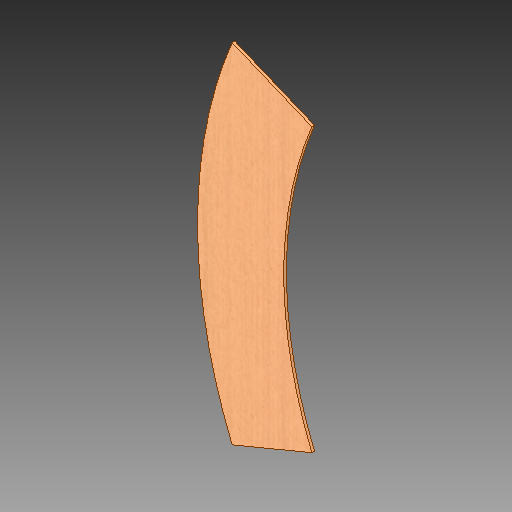
# Autodesk Inventor part: rearformer
Saved by Autodesk Inventor 2019 (Build 230136000, 136)
## iProperties
Created: 2019-01-07
Part Number: rearformer
Material: Wood (Cherry)
Document SubType Name: Modeling
Designer: gaincarlo
Density: 0.63 g/cm^3
Appearance: Cherry - Natural Low Gloss
Author: gaincarlo
Autodesk Inventor part; units mm, degrees
ref_plane "YZ Plane" through (0, 0, 0) normal (1, 0, 0) x (0, 1, 0)
ref_plane "XZ Plane" through (0, 0, 0) normal (0, 1, 0) x (-1, 0, 0)
ref_plane "Work Plane1" through (0, 0, 0) normal (0, 0, 1) x (1, 0, 0)
sketch "Sketch1" plane through (0, 0, 0) normal (0, 0, 1) x (1, 0, 0)
  line L0 (-300, -300) -> (-300, 300) construction
  line L1 (-300, 300) -> (300, 300) construction
  line L2 (300, 300) -> (300, -300) construction
  line L3 (300, -300) -> (-300, -300) construction
  line L4 (-254.3277, 283.4578) -> (-250.5009, 292.6966) construction
  line L5 (-250.5009, 292.6966) -> (303.8268, 63.0866) construction
  line L6 (303.8268, 63.0866) -> (300, 53.8478) construction
  line L7 (300, 53.8478) -> (-254.3277, 283.4578) construction
  line L8 (300, -53.8478) -> (303.8268, -63.0866) construction
  line L9 (303.8268, -63.0866) -> (-250.5009, -292.6966) construction
  line L10 (-250.5009, -292.6966) -> (-254.3277, -283.4578) construction
  line L11 (-254.3277, -283.4578) -> (300, -53.8478) construction
  line L12 (-254.3277, 283.4578) -> (-250.5009, 292.6966) construction
  line L13 (-250.5009, 292.6966) -> (303.8268, 63.0866) construction
  line L14 (303.8268, 63.0866) -> (300, 53.8478) construction
  line L15 (300, 53.8478) -> (-254.3277, 283.4578) construction
  line L16 (300, -53.8478) -> (303.8268, -63.0866) construction
  line L17 (303.8268, -63.0866) -> (-250.5009, -292.6966) construction
  line L18 (-250.5009, -292.6966) -> (-254.3277, -283.4578) construction
  line L19 (-254.3277, -283.4578) -> (300, -53.8478) construction
  arc A0 (34.4092, 161.6757) -> (34.4092, -161.6757) centre (430, 0) ccw construction
  line L20 (35.1767, 163.5412) -> (-57.2112, 201.8095)
  line L21 (35.1767, -163.5412) -> (-57.2112, -201.8095)
  arc A1 (35.1767, 163.5412) -> (35.1767, -163.5412) centre (430, 0) ccw
  arc A2 (-57.2112, 201.8095) -> (-57.2112, -201.8095) centre (430, 0) ccw
  point P0 (0, 0)
  dimension "d2" = 100
  constraints: 44 end point, 4 point on circle, 4 point on line, 2 centre point, 2 coincident, 2 horizontal, 2 vertical, 28 other
  measures "d2" radial gap between concentric circles of A2 A0
extrude "Extrusion1" add sketch "Sketch1" along normal blind 3
body "Solid1"
